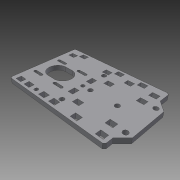
# Autodesk Inventor part: x_motor_back
Saved by Autodesk Inventor 2014 (Build 180170000, 170)
## iProperties
Created: 2013-11-30
Part Number: x_motor_back
Material: Generic
Document SubType Name: Modeling
Designer: buben
Density: 1 g/cm^3
Appearance: Anodized - Dark Gray
Author: buben
Subject: Laser Cutted
Autodesk Inventor part; units mm, degrees
ref_plane "YZ Plane" through (0, 0, 0) normal (1, 0, 0) x (0, 1, 0)
ref_plane "XZ Plane" through (0, 0, 0) normal (0, 1, 0) x (-1, 0, 0)
ref_plane "XY Plane" through (0, 0, 0) normal (0, 0, 1) x (1, 0, 0)
sketch "Sketch1" plane through (0, 0, 0) normal (0, 0, 1) x (1, 0, 0)
  line L0 (0, 0) -> (125, 0)
  line L1 (125, 86) -> (0, 86)
  line L2 (0, 86) -> (0, 0)
  line L3 (12.7, 55.5) -> (43.7, 55.5) construction
  line L4 (43.7, 55.5) -> (43.7, 24.5) construction
  line L5 (43.7, 24.5) -> (12.7, 24.5) construction
  line L6 (12.7, 24.5) -> (12.7, 55.5) construction
  line L7 (7.7, 55.5) -> (17.7, 55.5) construction
  line L8 (7.7, 53.8) -> (17.7, 53.8)
  line L9 (17.7, 57.2) -> (7.7, 57.2)
  arc A0 (7.7, 57.2) -> (7.7, 53.8) centre (7.7, 55.5) ccw
  arc A1 (17.7, 53.8) -> (17.7, 57.2) centre (17.7, 55.5) ccw
  line L10 (38.7, 55.5) -> (48.7, 55.5) construction
  line L11 (38.7, 53.8) -> (48.7, 53.8)
  line L12 (48.7, 57.2) -> (38.7, 57.2)
  arc A2 (38.7, 57.2) -> (38.7, 53.8) centre (38.7, 55.5) ccw
  arc A3 (48.7, 53.8) -> (48.7, 57.2) centre (48.7, 55.5) ccw
  line L13 (7.7, 24.5) -> (17.7, 24.5) construction
  line L14 (7.7, 22.8) -> (17.7, 22.8)
  line L15 (17.7, 26.2) -> (7.7, 26.2)
  arc A4 (7.7, 26.2) -> (7.7, 22.8) centre (7.7, 24.5) ccw
  arc A5 (17.7, 22.8) -> (17.7, 26.2) centre (17.7, 24.5) ccw
  line L16 (38.7, 24.5) -> (48.7, 24.5) construction
  line L17 (38.7, 26.2) -> (48.7, 26.2)
  line L18 (48.7, 22.8) -> (38.7, 22.8)
  arc A6 (38.7, 26.2) -> (38.7, 22.8) centre (38.7, 24.5) ccw
  arc A7 (48.7, 22.8) -> (48.7, 26.2) centre (48.7, 24.5) ccw
  line L19 (23.2, 40) -> (33.2, 40) construction
  line L20 (23.2, 51.5) -> (33.2, 51.5)
  line L21 (33.2, 28.5) -> (23.2, 28.5)
  arc A8 (23.2, 51.5) -> (23.2, 28.5) centre (23.2, 40) ccw
  arc A9 (33.2, 28.5) -> (33.2, 51.5) centre (33.2, 40) ccw
  line L22 (6, 77) -> (14, 77)
  line L23 (14, 77) -> (14, 71)
  line L24 (14, 71) -> (6, 71)
  line L25 (6, 71) -> (6, 77)
  line L26 (6, 9) -> (14, 9)
  line L27 (14, 9) -> (14, 3)
  line L28 (14, 3) -> (6, 3)
  line L29 (6, 3) -> (6, 9)
  line L30 (125, 71) -> (135, 61)
  line L31 (135, 61) -> (135, 19)
  line L32 (135, 19) -> (125, 9)
  line L33 (125, 0) -> (125, 9)
  line L34 (125, 71) -> (125, 86)
  line L35 (72, 63) -> (80, 63)
  line L36 (80, 63) -> (80, 57)
  line L37 (80, 57) -> (72, 57)
  line L38 (72, 57) -> (72, 63)
  line L39 (72, 23) -> (80, 23)
  line L40 (80, 23) -> (80, 17)
  line L41 (80, 17) -> (72, 17)
  line L42 (72, 17) -> (72, 23)
  line L43 (0, 67) -> (129, 67) construction
  line L44 (0, 13) -> (129, 13) construction
  line L45 (129, 67) -> (129, 13) construction
  line L46 (17, 83) -> (25, 83)
  line L47 (25, 83) -> (25, 77)
  line L48 (25, 77) -> (17, 77)
  line L49 (17, 77) -> (17, 83)
  line L50 (113, 77) -> (121, 77)
  line L51 (121, 77) -> (121, 71)
  line L52 (121, 71) -> (113, 71)
  line L53 (113, 71) -> (113, 77)
  line L54 (113, 9) -> (121, 9)
  line L55 (121, 9) -> (121, 3)
  line L56 (121, 3) -> (113, 3)
  line L57 (113, 3) -> (113, 9)
  circle A10 centre (128, 60) radius 2.75
  circle A11 centre (63, 67) radius 2.75
  circle A12 centre (63, 13) radius 2.75
  circle A13 centre (128, 20) radius 2.75
  line L58 (57, 86) -> (57, 0) construction
  line L59 (11.7, 61.5) -> (54.7, 61.5) construction
  line L60 (54.7, 61.5) -> (54.7, 18.5) construction
  line L61 (54.7, 18.5) -> (11.7, 18.5) construction
  line L62 (11.7, 18.5) -> (11.7, 61.5) construction
  line L63 (17.7, 24.5) -> (48.7, 24.5) construction
  line L64 (110, 63) -> (118, 63)
  line L65 (118, 63) -> (118, 57)
  line L66 (118, 57) -> (110, 57)
  line L67 (110, 57) -> (110, 63)
  line L68 (110, 23) -> (118, 23)
  line L69 (118, 23) -> (118, 17)
  line L70 (118, 17) -> (110, 17)
  line L71 (110, 17) -> (110, 23)
  line L72 (85, 77) -> (93, 77)
  line L73 (93, 77) -> (93, 71)
  line L74 (93, 71) -> (85, 71)
  line L75 (85, 71) -> (85, 77)
  line L76 (85, 9) -> (93, 9)
  line L77 (93, 9) -> (93, 3)
  line L78 (93, 3) -> (85, 3)
  line L79 (85, 3) -> (85, 9)
  line L80 (57, 77) -> (65, 77)
  line L81 (65, 77) -> (65, 71)
  line L82 (65, 71) -> (57, 71)
  line L83 (57, 71) -> (57, 77)
  line L84 (57, 9) -> (65, 9)
  line L85 (65, 9) -> (65, 3)
  line L86 (65, 3) -> (57, 3)
  line L87 (57, 3) -> (57, 9)
  line L88 (68, 83) -> (76, 83)
  line L89 (76, 83) -> (76, 77)
  line L90 (76, 77) -> (68, 77)
  line L91 (68, 77) -> (68, 83)
  line L92 (96, 83) -> (104, 83)
  line L93 (104, 83) -> (104, 77)
  line L94 (104, 77) -> (96, 77)
  line L95 (96, 77) -> (96, 83)
  circle A14 centre (71, 40) radius 5 construction
  circle A15 centre (103, 40) radius 5 construction
  circle A16 centre (103, 40) radius 2.75
  circle A17 centre (71, 40) radius 2.75
  point P0 (28.2, 40)
  point P1 (28.2, 55.5)
  point P2 (12.7, 40)
  point P3 (129, 40)
  point P4 (11.7, 40)
  point P5 (33.2, 24.5)
  point P6 (33.2, 18.5)
  dimension "d1" = 31
  dimension "d2" = 31
  dimension "d3" = 3.4
  dimension "d4" = 3.4
  dimension "d5" = 3.4
  dimension "d6" = 3.4
  dimension "d7" = 10
  dimension "d8" = 23
  dimension "d9" = 3
  dimension "d10" = 6
  dimension "d11" = 6
  dimension "d12" = 9
  dimension "d13" = 45
  dimension "d14" = 10
  dimension "d15" = 8
  dimension "d16" = 6
  dimension "d17" = 8
  dimension "d18" = 6
  dimension "d19" = 4
  dimension "d21" = 8
  dimension "d22" = 8
  dimension "d23" = 7.7
  dimension "d25" = 8
  dimension "d26" = 6
  dimension "d27" = 3
  dimension "d28" = 6
  dimension "d29" = 8
  dimension "d30" = 4
  dimension "d31" = 4
  dimension "d32" = 125
  dimension "d33" = 5.5
  dimension "d34" = 5.5
  dimension "d35" = 5.5
  dimension "d36" = 5.5
  dimension "d37" = 7
  dimension "d38" = 11
  dimension "d39" = 7
  dimension "d40" = 11
  dimension "d41" = 62
  dimension "d42" = 68
  dimension "d43" = 43
  dimension "d44" = 43
  dimension "d45" = 8
  dimension "d47" = 8
  dimension "d48" = 10
  dimension "d49" = 8
  dimension "d50" = 20
  dimension "d51" = 8
  dimension "d52" = 20
  dimension "d53" = 8
  dimension "d54" = 8
  dimension "d55" = 3
  dimension "d56" = 3
  dimension "d57" = 15
  dimension "d58" = 10
  dimension "d59" = 10
  dimension "d60" = 5.5
  dimension "d61" = 5.5
  dimension "d62" = 14
  dimension "d63" = 32
  dimension "d69" = 34
  constraints: 202 end point, 49 parallel, 33 collinear, 23 perpendicular, 20 point on circle, 20 tangent, 18 centre point, 18 horizontal, 11 midpoint, 8 point on line, 7 horizontal alignment, 6 coincident, 4 equal length, 3 vertical alignment
  measures "d1" distance of L3.start L3.end
  measures "d2" distance of L3.end L4.end
  measures "d3" distance between parallel lines of L8 L9
  measures "d4" distance between parallel lines of L11 L12
  measures "d5" distance between parallel lines of L14 L15
  measures "d6" distance between parallel lines of L18 L17
  measures "d7" distance of L7.start L7.end
  measures "d8" distance between parallel lines of L21 L20
  measures "d9" distance between parallel lines of L0 L28
  measures "d10" distance of L28.end L26.start
  measures "d11" distance of L24.end L22.start
  measures "d12" distance between parallel lines of L22 L1
  measures "d13" angle of L30 L34
  measures "d14" distance between parallel lines of L34 L31
  measures "d15" distance between parallel lines of L35 L24
  measures "d16" distance of L35.end L36.end
  measures "d17" distance between parallel lines of L41 L26
  measures "d18" distance of L39.end L40.end
  measures "d19" distance between parallel lines of L43 L24
  measures "d21" distance of L22.start L22.end
  measures "d22" distance of L27.end L28.end
  measures "d23" distance from line of L2 L7.start
  measures "d25" distance of L46.start L46.end
  measures "d26" distance of L48.end L46.start
  measures "d27" distance between parallel lines of L23 L49
  measures "d28" distance between parallel lines of L2 L29
  measures "d29" distance between parallel lines of L51 L53
  measures "d30" distance between parallel lines of L34 L51
  measures "d31" distance between parallel lines of L44 L26
  measures "d32" distance of L0.start L0.end
  measures "d33" diameter of A13
  measures "d34" diameter of A10
  measures "d35" diameter of A11
  measures "d36" diameter of A12
  measures "d37" distance from line of L31 A10.centre
  measures "d38" vertical distance of A10.centre L30.start
  measures "d39" distance from line of L31 A13.centre
  measures "d40" vertical distance of L32.end A13.centre
  measures "d41" distance from line of L34 A11.centre
  measures "d42" distance between parallel lines of L33 L58
  measures "d43" distance of L59.start L59.end
  measures "d44" distance of L61.end L59.start
  measures "d45" distance of L36.end L37.end
  measures "d47" distance of L64.start L64.end
  measures "d48" distance from line of A10.centre L65
  measures "d49" distance of L72.start L72.end
  measures "d50" distance between parallel lines of L53 L73
  measures "d51" distance of L80.start L80.end
  measures "d52" distance between parallel lines of L75 L81
  measures "d53" distance of L88.start L88.end
  measures "d54" distance of L92.start L92.end
  measures "d55" distance between parallel lines of L81 L91
  measures "d56" distance between parallel lines of L73 L95
  measures "d57" distance between parallel lines of L58 L38
  measures "d58" diameter of A14
  measures "d59" diameter of A15
  measures "d60" diameter of A17
  measures "d61" diameter of A16
  measures "d62" distance from line of L58 A14.centre
  measures "d63" distance from line of L31 A15.centre
  measures "d69" distance between parallel lines of L39 L37
extrude "Extrusion1" add sketch "Sketch1" along normal blind 6
chamfer "Chamfer1" distance 2 angle 45 4 edges at (0, 0, 3) (125, 0, 3) (125, 86, 3) (0, 86, 3)
sketch "Sketch2" plane through (0, 0, 6) normal (0, 0, 1) x (1, 0, 0)
  arc A0 (33.2, 28.5) -> (33.2, 51.5) centre (33.2, 40) ccw projected
  line L0 (14, 9) -> (14, 3) projected
  line L1 (14, 3) -> (6, 3) projected
  line L2 (6, 9) -> (14, 9) projected
  circle A1 centre (71, 40) radius 2.75 projected
  line L3 (0, 84) -> (0, 2) projected
  line L4 (11.7, 61.5) -> (54.7, 61.5) construction
  line L5 (54.7, 61.5) -> (54.7, 18.5) construction
  line L6 (54.7, 18.5) -> (11.7, 18.5) construction
  line L7 (11.7, 18.5) -> (11.7, 61.5) construction
  line L8 (19.5, 9) -> (27.5, 9)
  line L9 (27.5, 9) -> (27.5, 3)
  line L10 (27.5, 3) -> (19.5, 3)
  line L11 (19.5, 3) -> (19.5, 9)
  line L12 (42.5, 9) -> (50.5, 9)
  line L13 (50.5, 9) -> (50.5, 3)
  line L14 (50.5, 3) -> (42.5, 3)
  line L15 (42.5, 3) -> (42.5, 9)
  line L16 (27.5, 9) -> (42.5, 3) construction
  line L17 (27.5, 3) -> (42.5, 9) construction
  circle A2 centre (35, 6) radius 2.25
  line L18 (58, 55.5) -> (64, 55.5)
  line L19 (64, 55.5) -> (64, 47.5)
  line L20 (64, 47.5) -> (58, 47.5)
  line L21 (58, 47.5) -> (58, 55.5)
  line L22 (58, 32.5) -> (64, 32.5)
  line L23 (64, 32.5) -> (64, 24.5)
  line L24 (64, 24.5) -> (58, 24.5)
  line L25 (58, 24.5) -> (58, 32.5)
  line L26 (58, 47.5) -> (64, 32.5) construction
  line L27 (58, 32.5) -> (64, 47.5) construction
  circle A3 centre (71, 40) radius 5 construction
  circle A4 centre (61, 40) radius 4.5 construction
  circle A5 centre (61, 40) radius 2.25
  point P0 (0, 0)
  point P1 (54.7, 40)
  point P2 (33.2, 61.5)
  dimension "d71" = 43
  dimension "d72" = 43
  dimension "d73" = 8
  dimension "d74" = 8
  dimension "d75" = 15
  dimension "d76" = 4.5
  dimension "d78" = 21
  dimension "d79" = 8
  dimension "d80" = 8
  dimension "d81" = 6
  dimension "d82" = 15
  dimension "d84" = 58
  dimension "d85" = 10
  dimension "d86" = 9
  dimension "d87" = 4.5
  constraints: 48 end point, 10 parallel, 6 collinear, 5 horizontal, 5 midpoint, 5 perpendicular, 4 centre point, 3 coincident, 2 horizontal alignment, 1 vertical alignment
  measures "d71" distance of L4.end L5.end
  measures "d72" distance of L5.end L6.end
  measures "d73" distance of L8.start L8.end
  measures "d74" distance of L12.start L12.end
  measures "d75" distance between parallel lines of L15 L9
  measures "d76" diameter of A2
  measures "d78" distance from line of A2.centre L0
  measures "d79" distance of L20.end L18.start
  measures "d80" distance of L24.end L22.start
  measures "d81" distance of L18.start L18.end
  measures "d82" distance between parallel lines of L22 L20
  measures "d84" distance between parallel lines of L3 L21
  measures "d85" diameter of A3
  measures "d86" diameter of A4
  measures "d87" diameter of A5
extrude "Extrusion2" cut sketch "Sketch2" against normal through all contours L8 L9 L10 L11 | L12 L13 L14 L15 | A2 | L18 L19 L20 L21 | L22 L23 L24 L25 | A5
body "Solid1"
